Autodesk Fusion 360 part; units mm, degrees
(part 2 of 2)
chamfer "Chamfer38" distance 25 angle 65 1 edges at (5, -0.75, 6.25) measured on face at (75.2333, -0.5833, 6.25) on bodies 3
chamfer "Chamfer39" distance 53.6 angle 25 1 edges at (5, -0.75, 113.57) measured on face at (5, -0.9167, 77.7651) on bodies 3
chamfer "Chamfer40" distance 25 angle 65 1 edges at (110.35, -0.75, 113.57) measured on face at (118.1167, 11.4167, 113.57) on bodies 3
chamfer "Chamfer41" distance 53.6 angle 25 1 edges at (110.35, -0.75, 6.25) measured on face at (110.35, -0.9167, 42.0549) on bodies 3
chamfer "Chamfer42" distance 25 angle 65 1 edges at (110.1, 17.75, 6.25) measured on face at (56.7, 17.5833, 6.25) on bodies 3
chamfer "Chamfer43" distance 53.6 angle 25 1 edges at (110.1, 17.75, 113.57) measured on face at (110.1, 17.9167, 77.7651) on bodies 3
extrude "Extrude78" add 1 faces at (127.3, 18.25, 59.8942) along direction (0, 1, 0) blind 0.5 on bodies 3 bodies 3
extrude "Extrude79" add 1 faces at (127.3833, -1.25, 59.9258) along direction (0, -1, 0) blind 0.5 on bodies 3 bodies 3
hidden bodies 1
named bodies: "NES Cart"
